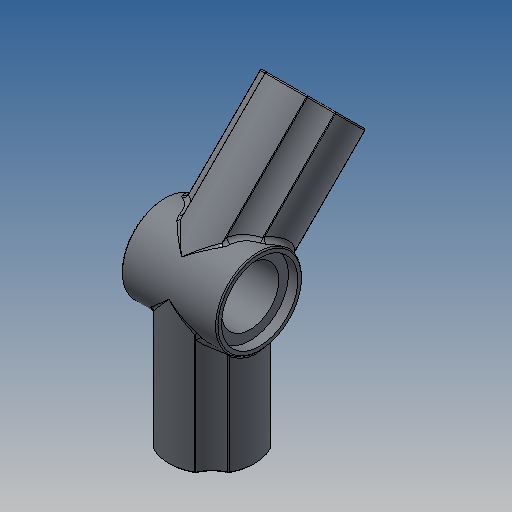
# Autodesk Inventor part: 32192-Red
Saved by Autodesk Inventor 2025 (Build 290162010, 162A)
## iProperties
Created: 2002-08-04
Part Number: 32192-Red
Material: ABS Plastic
Document SubType Name: Modellieren
Designer: D. Kohfeld
Density: 1.06 g/cm^3
Appearance: LtBluishGray
Mass: 0.687316 g
Surface Area: 10.5462 cm^2
Volume: 0.648411 cm^3
Control State: 0
Master: False
Checked Out: False
Shininess: 20.0
Angle Display Precision: 2
Document Length Units: 11269
Document Angle Units: 11279
Document Time Units: 11290
Document Mass Units: 11283
Document Length Units Precision: 3
Document Angle Units Precision: 2
Density: 0.0
Volumn: 0.0
Area: 0.0
PropertySet Name: Model Information
Author: D. Kohfeld
Autodesk Inventor part; units mm, degrees
ref_plane "YZ Plane" through (0, 0, 0) normal (1, 0, 0) x (0, 1, 0)
ref_plane "XZ Plane" through (0, 0, 0) normal (0, 1, 0) x (-1, 0, 0)
ref_plane "XY Plane" through (0, 0, 0) normal (0, 0, 1) x (1, 0, 0)
sketch "Skizze1" plane through (0, 0, 0) normal (0, 0, 1) x (1, 0, 0)
  arc A0 (-3.141014, 1.758986) -> (-1.758986, 3.141014) centre (-4, 4) ccw
  arc A1 (-1.758986, -3.141014) -> (-3.141014, -1.758986) centre (-4, -4) ccw
  arc A2 (3.141014, -1.758986) -> (1.758986, -3.141014) centre (4, -4) ccw
  arc A3 (1.758986, 3.141014) -> (3.141014, 1.758986) centre (4, 4) ccw
  line L0 (4, 4) -> (-4, 4) construction
  line L1 (-4, 4) -> (-4, -4) construction
  arc A4 (-3.141014, 1.758986) -> (-3.141014, -1.758986) centre (0, 0) ccw
  arc A5 (-1.758986, -3.141014) -> (1.758986, -3.141014) centre (0, 0) ccw
  arc A6 (3.141014, -1.758986) -> (3.141014, 1.758986) centre (0, 0) ccw
  arc A7 (1.758986, 3.141014) -> (-1.758986, 3.141014) centre (0, 0) ccw
  circle A8 centre (0, 0) radius 2.4 construction
  line L2 (-0.8, 2.262742) -> (-0.8, 0.8)
  line L3 (-0.8, 0.8) -> (-2.262742, 0.8)
  line L4 (-2.262742, -0.8) -> (-0.8, -0.8)
  line L5 (-0.8, -0.8) -> (-0.8, -2.262742)
  line L6 (0.8, -2.262742) -> (0.8, -0.8)
  line L7 (0.8, -0.8) -> (2.262742, -0.8)
  line L8 (2.262742, 0.8) -> (0.8, 0.8)
  line L9 (0.8, 0.8) -> (0.8, 2.262742)
  arc A9 (0.8, 2.262742) -> (-0.8, 2.262742) centre (0, 0) ccw
  arc A10 (-2.262742, 0.8) -> (-2.262742, -0.8) centre (0, 0) ccw
  arc A11 (-0.8, -2.262742) -> (0.8, -2.262742) centre (0, 0) ccw
  arc A12 (2.262742, -0.8) -> (2.262742, 0.8) centre (0, 0) ccw
  point P0 (0, 4)
  point P1 (-4, 0)
  dimension "d50" = 4.8
  dimension "d46" = 8
  dimension "d48" = 2.4
  dimension "d49" = 7.2
  dimension "d51" = 1.6
  constraints: 24 point on circle, 20 end point, 12 centre point, 8 equal length, 4 parallel, 4 perpendicular, 3 concentric, 3 equal radius, 2 coincident, 2 horizontal alignment, 2 midpoint, 2 vertical alignment, 1 horizontal, 1 vertical, 14 other
  measures "d46" distance of L0.start L0.end
  measures "d48" radius of A0
  measures "d49" diameter of A4
  measures "d51" distance between parallel lines of L9 L2
extrude "Extrusion1" add sketch "Skizze1" against normal blind 12 contours A0 A7 A3 A6 A2 A5 A1 A4 | A9 L9 L8 A12 L7 L6 A11 L5 L4 A10 L3 L2
sketch "Sketch20" plane through (0, 0, -12) normal (0, 0, -1) x (-1, 0, 0)
  arc A0 (-1.758986, -3.141014) -> (1.758986, -3.141014) centre (0, 0) ccw
  circle A1 centre (0, 0) radius 2.4
  line L0 (-0.8, 2.262742) -> (-0.8, 0.8)
  line L1 (-0.8, 0.8) -> (-2.262742, 0.8)
  line L2 (-2.262742, -0.8) -> (-0.8, -0.8)
  line L3 (-0.8, -0.8) -> (-0.8, -2.262742)
  line L4 (0.8, -2.262742) -> (0.8, -0.8)
  line L5 (0.8, -0.8) -> (2.262742, -0.8)
  line L6 (2.262742, 0.8) -> (0.8, 0.8)
  line L7 (0.8, 0.8) -> (0.8, 2.262742)
  dimension "d60" = 4.8
  dimension "d63" = 1.6
  constraints: 16 end point, 7 equal length, 4 perpendicular, 3 parallel, 1 coincident, 1 vertical, 10 other
  measures "d63" distance between parallel lines of L7 L0
extrude "Extrusion15" cut sketch "Sketch20" against normal blind 8 contours A1 L5 L4 L3 L2 L1 L0 L7 L6
extrude "Extrusion16" cut sketch "Sketch20" against normal blind 0.4
pattern_circular "Circular Pattern1" count 2 over 135 about axis through (-10, 0, 0) along (1, 0, 0) of "Extrusion1", "Extrusion15", "Extrusion16"
sketch "Sketch6" plane through (0, 0, 0) normal (1, 0, 0) x (0, 1, 0)
  circle A0 centre (0, 0) radius 3.6
  dimension "d8" = 7.2
  constraints: 3 coincident, 1 centre point
  measures "d8" diameter of A0
extrude "Extrusion4" add sketch "Sketch6" along normal mid plane 8
sketch "Sketch12" plane through (4, 0, 0) normal (1, 0, 0) x (0, 0, -1)
  circle A0 centre (0, 0) radius 3.6 projected
  constraints: 1 coincident
hole "Hole1" at (4, 0, 0) direction (-1, 0, 0) diameter 4.8 depth 8 counterbore diameter 6.4 counterbore depth 0.8
sketch "Sketch13" plane through (-4, 0, 0) normal (-1, 0, 0) x (0, 0, 1)
  circle A0 centre (0, 0) radius 2.4 projected
  circle A1 centre (0, 0) radius 3.2 projected
extrude "Extrusion9" cut sketch "Sketch13" against normal blind 0.8
fillet "Fillet1" radius 0.4 23 edges at (2.2073, -2.4043, -2.6794) (3.6, 0, -3.6) (2.2073, 2.4043, -2.6794) (-2.2073, 2.4043, -2.6794) (-3.6, 0, -3.6) (-2.2073, -2.4043, -2.6794) (2.5434, 3.551, 0.5917) (1.8854, 3.5673, -0.4843) (0, 3.6, -1.4912) (3.6, 2.5456, 2.5456) (-2.5434, 3.551, 0.5917) (-1.8854, 3.5673, -0.4843) (-3.6, 2.5456, 2.5456) (-2.2073, 0.1945, 3.5947) (2.2073, 0.1945, 3.5947) (0.9089, -3.4834, -0.9089) (-0.9089, -3.4834, -0.9089) (0.9089, -1.8204, 3.1058) (-0.9089, -1.8204, 3.1058) (1.571, 3.4013, -1.1795) (1.571, 3.2391, -1.571) (-1.571, 3.2391, -1.571) (-1.571, 3.4013, -1.1795)
fillet "Fillet1" radius 0.1 34 edges at (-1.759, -3.141, -6.8795) (-3.141, -1.759, -7.5705) (1.759, -3.141, -6.8795) (3.141, -1.759, -7.5705) (4, -3.6, 0) (-4, -3.6, 0) (3.141, 1.759, -7.5705) (1.759, 3.141, -6.8795) (-1.759, 3.141, -6.8795) (-3.141, 1.759, -7.5705) (3.141, 4.1094, 6.5969) (1.759, 2.6435, 7.0856) (-1.759, 2.6435, 7.0856) (-3.141, 4.1094, 6.5969) (-3.141, 6.5969, 4.1094) (-1.759, 7.0856, 2.6435) (1.759, 7.0856, 2.6435) (3.141, 6.5969, 4.1094) (0, 5.9397, 11.0309) (-2.3029, 6.8569, 10.1137) (-3.6, 8.4853, 8.4853) (0, -3.6, -12) (-2.3029, -2.3029, -12) (-3.6, 0, -12) (-2.3029, 2.3029, -12) (0, 3.6, -12) (2.3029, 2.3029, -12) (3.6, 0, -12) (2.3029, -2.3029, -12) (2.3029, 6.8569, 10.1137) (3.6, 8.4853, 8.4853) (2.3029, 10.1137, 6.8569) (0, 11.0309, 5.9397) (-2.3029, 10.1137, 6.8569)
equation "\"d50\" = kd"
equation "\"d46\" = lu"
equation "\"d48\" = 0.5 * kd"
equation "\"d49\" = tlad"
equation "\"d51\" = axlet"
equation "\"ht\" = 1.5 * lu"
equation "\"d60\" = kd"
equation "\"d63\" = axlet"
equation "\"d61\" = lu"
equation "\"d8\" = tlad"
equation "\"d9\" = lu"
equation "\"d24\" = tpd"
equation "\"d26\" = tsd"
equation "\"d27\" = tsl"
equation "\"d29\" = lu"
equation "\"d32\" = tsl"
equation "\"kd\" = 4.8"
equation "\"lu\" = 8"
equation "\"tlad\" = 7.2"
equation "\"axlet\" = 1.6"
equation "\"tpd\" = 4.8"
equation "\"tsd\" = 6.4"
equation "\"tsl\" = 0.8"
body "Solid1"
